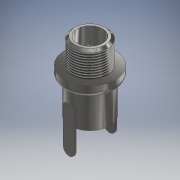
# Autodesk Inventor part: Plug alimentation
Saved by Autodesk Inventor 2017 (Build 210142000, 142)
## iProperties
Company: FABLAB Frenchmakers
Part Number: Plug alimentation
Project: 1420 VAUBAN 3D XL
Material: ----------
Catalog Web Link: http://www.frenchmakers.com/
Document SubType Name: Modeling
Designer: FABLAB Frenchmakers
Mass: 5.41927 g
Surface Area: 9.22137 cm^2
Volume: 0.689475 cm^3
Density: 7.86 g/cm^3
Appearance: Acier - Poli
Stock Number: 1420-09-01
Autodesk Inventor part; units mm, degrees
ref_plane "YZ Plane" through (0, 0, 0) normal (1, 0, 0) x (0, 1, 0)
ref_plane "XZ Plane" through (0, 0, 0) normal (0, 1, 0) x (-1, 0, 0)
ref_plane "XY Plane" through (0, 0, 0) normal (0, 0, 1) x (1, 0, 0)
sketch "Esquisse1" plane through (0, 0, 0) normal (0, 0, 1) x (1, 0, 0)
  circle A0 centre (0, 0) radius 3.775
  dimension "d0" = 7.55
  constraints: 1 centre point, 1 coincident
  measures "d0" diameter of A0
extrude "Extrusion1" add sketch "Esquisse1" along normal blind 5.5
sketch "Esquisse2" plane through (0, 0, 0) normal (0, 0, -1) x (-1, 0, 0)
  circle A0 centre (0, 0) radius 5.5
  dimension "d3" = 11
  constraints: 1 centre point, 1 coincident
  measures "d3" diameter of A0
extrude "Extrusion2" add sketch "Esquisse2" along normal blind 2.3
sketch "Esquisse3" plane through (0, 0, -2.3) normal (0, 0, -1) x (-1, 0, 0)
  circle A0 centre (0, 0) radius 4.25
  dimension "d6" = 8.5
  constraints: 1 centre point, 1 coincident
  measures "d6" diameter of A0
extrude "Extrusion3" add sketch "Esquisse3" along normal blind 7
fillet "Congé1" radius 1 1 edges at (5.5, 0, -2.3)
sketch "Esquisse4" plane through (0, 0, 5.5) normal (0, 0, 1) x (1, 0, 0)
  circle A0 centre (0, 0) radius 2.75
  dimension "d10" = 5.5
  constraints: 1 centre point, 1 coincident
  measures "d10" diameter of A0
extrude "Extrusion4" cut sketch "Esquisse4" against normal blind 9
sketch "Esquisse5" plane through (0, 0, -3.5) normal (0, 0, 1) x (1, 0, 0)
  circle A0 centre (0, 0) radius 1.2
  dimension "d13" = 2.4
  constraints: 1 centre point, 1 coincident
  measures "d13" diameter of A0
extrude "Extrusion5" add sketch "Esquisse5" along normal blind 7.2
fillet "Congé2" radius 1.2 1 edges at (-1.2, 0, 3.7)
thread "Filetage1" size "M8x0.5" class "6g" standard "ISO Metric profile" full length
sketch "Esquisse6" plane through (0, 0, 0) normal (1, 0, 0) x (0, 1, 0)
  line L0 (4.25, -14.8) -> (4.25, -5.8)
  line L1 (4.25, -5.8) -> (4.05, -5.8)
  line L2 (4.05, -5.8) -> (4.05, -5.5)
  line L3 (4.05, -5.5) -> (4.55, -5.5)
  line L4 (4.55, -5.5) -> (4.55, -14.8)
  line L5 (4.55, -14.8) -> (4.25, -14.8)
  line L6 (4.25, -2.3) -> (4.25, -9.3) projected
  line L7 (4.25, -2.3) -> (-4.25, -2.3) projected
  point P0 (0, 0)
  dimension "d19" = 0.3
  dimension "d20" = 0.3
  dimension "d21" = 9.3
  dimension "d22" = 3.2
  dimension "d24" = 0.2
  constraints: 12 end point, 5 perpendicular, 1 point on line, 1 vertical
  measures "d19" distance between parallel lines of L4 L0
  measures "d20" distance of L1.end L2.end
  measures "d21" distance of L3.end L4.end
  measures "d22" distance between parallel lines of L7 L3
  measures "d24" distance between parallel lines of L0 L2
extrude "Extrusion6" add sketch "Esquisse6" along normal mid plane 2.5
fillet "Congé3" radius 1.25 2 edges at (1.25, 4.4, -14.8) (-1.25, 4.4, -14.8)
pattern_circular "Réseau circulaire1" count 3 over 180 about axis through (0, 0, -10) along (0, 0, 1) of "Extrusion6", "Congé3"
chamfer "Chanfrein1" distance 0.5 angle 45 1 edges at (-3.775, 0, 5.5)
